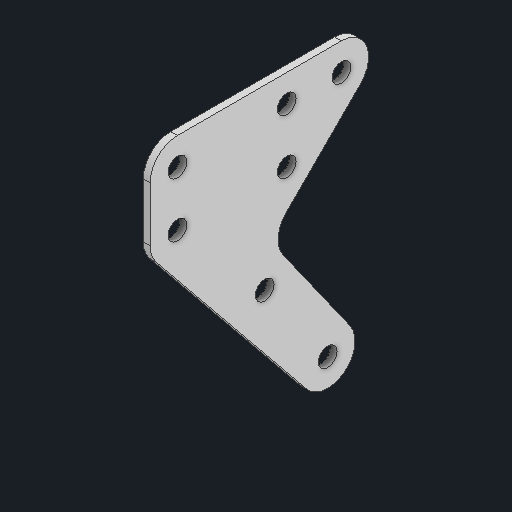
# Autodesk Inventor part: triangle_brace_gusset
Saved by Autodesk Inventor 2025 (Build 290162000, 162)
## iProperties
Created: 2024-10-13
Part Number: triangle_brace_gusset
Material: Generic
Document SubType Name: Modeling
Designer: Averey Ku
Density: 1 g/cm^3
Appearance: Default
d0: 0.500 in
d1: 0.500 in
d4: 0.250 in
d6: 0.172 in
Author: Averey Ku
Autodesk Inventor part; units mm, degrees
ref_plane "YZ Plane" through (0, 0, 0) normal (1, 0, 0) x (0, 1, 0)
ref_plane "XZ Plane" through (0, 0, 0) normal (0, 1, 0) x (-1, 0, 0)
ref_plane "XY Plane" through (0, 0, 0) normal (0, 0, 1) x (1, 0, 0)
sketch "maiin" plane through (0, 0, 0) normal (0, 0, 1) x (1, 0, 0)
  arc A0 (6.5899, -1.511) -> (-1.5658, -0.8125) centre (2.0978, -5.9991) ccw
  circle A1 centre (-6.5018, 3.4753) radius 2.1844
  line L0 (-31.2537, -6.2516) -> (11.7059, 28.671)
  line L1 (-23.5847, -16.3655) -> (-1.5658, -0.8125)
  circle A2 centre (-27.2482, -11.1789) radius 2.1844
  arc A3 (-31.2537, -6.2516) -> (-23.5847, -16.3655) centre (-27.2482, -11.1789) ccw
  circle A4 centre (28.4, -14.3563) radius 2.1844
  line L2 (34.75, -14.3563) -> (34.75, 23.7437)
  line L3 (15.7114, 30.0937) -> (28.4, 30.0937)
  circle A5 centre (28.4, 23.7437) radius 2.1844
  circle A6 centre (28.4, -1.6563) radius 2.1844
  arc A7 (23.9079, -18.8444) -> (34.75, -14.3563) centre (28.4, -14.3563) ccw
  line L4 (23.9079, -18.8444) -> (6.5899, -1.511)
  circle A8 centre (15.7114, 23.7437) radius 2.1844
  circle A9 centre (15.7114, -1.6563) radius 2.1844
  arc A10 (34.75, 23.7437) -> (28.4, 30.0937) centre (28.4, 23.7437) ccw
  arc A11 (15.7114, 30.0937) -> (11.7059, 28.671) centre (15.7114, 23.7437) ccw
  point P0 (10.0881, 4.3711)
  dimension "d0" = 12.7
  dimension "d1" = 12.7
  dimension "d4" = 6.35
  dimension "d6" = 4.3688
  measures "d0" diameter of A3
  measures "d1" diameter of A7
  measures "d4" radius of A0
  measures "d6" diameter of A9
sketch "Sketch1" plane through (0, 0, 0) normal (1, 0, 0) x (0, 1, 0)
  arc A0 (-21.8101, -25.2546) -> (-29.9658, -24.5561) centre (-26.3022, -29.7428) ccw
  circle A1 centre (-34.9019, -20.2684) radius 2.1844
  line L0 (-59.6538, -29.9953) -> (-16.6941, 4.9273)
  line L1 (-51.9847, -40.1092) -> (-29.9658, -24.5561)
  circle A2 centre (-55.6483, -34.9226) radius 2.1844
  arc A3 (-59.6538, -29.9953) -> (-51.9847, -40.1092) centre (-55.6483, -34.9226) ccw
  circle A4 centre (0, -38.1) radius 2.1844
  line L2 (6.35, -38.1) -> (6.35, 0)
  line L3 (-12.6886, 6.35) -> (0, 6.35)
  circle A5 centre (0, 0) radius 2.1844
  circle A6 centre (0, -25.4) radius 2.1844
  arc A7 (-4.4921, -42.5881) -> (6.35, -38.1) centre (0, -38.1) ccw
  line L4 (-4.4921, -42.5881) -> (-21.8101, -25.2546)
  circle A8 centre (-12.6886, 0) radius 2.1844
  circle A9 centre (-12.6886, -25.4) radius 2.1844
  arc A10 (6.35, 0) -> (0, 6.35) centre (0, 0) ccw
  arc A11 (-12.6886, 6.35) -> (-16.6941, 4.9273) centre (-12.6886, 0) ccw
  constraints: 1 other
extrude "Extrusion1" add sketch "Sketch1" along normal blind 1.5875
body "Solid1"
